Autodesk Fusion 360 part; units mm, degrees
note: some values were not read from the file. Chosen so that the rebuilt part matches the saved one: which face or edge a step refers to. Set by a fixed rule: which sketch regions a step uses.
(part 3 of 7)
  spline S225 degree 3 poles (8.0112, 79.2711) (8.0608, 79.0575) (8.1057, 78.8514) (8.1464, 78.6528) knots 0 0 0 0 1 1 1 1
  spline S226 degree 3 poles (0.8014, 82.2545) (1.2067, 81.299) (1.5221, 80.4293) (1.767, 79.6553) knots 0 0 0 0 1 1 1 1
  arc A227 (1.9503, 79.0495) -> (2.3228, 78.7606) centre (2.3346, 79.1604) ccw
  spline S227 degree 3 poles (4.2579, 78.9588) (4.3292, 79.1486) (4.4058, 79.3452) (4.4881, 79.5484) knots 0 0 0 0 1 1 1 1
  arc A228 (7.2526, 81.938) -> (5.6547, 82.0638) centre (0, 0) ccw
  spline S228 degree 3 poles (-1.9503, 79.0495) (-1.8941, 79.2443) (-1.8331, 79.4462) (-1.767, 79.6553) knots 0 0 0 0 1 1 1 1
  spline S229 degree 3 poles (1.767, 79.6553) (1.8331, 79.4462) (1.8941, 79.2443) (1.9503, 79.0495) knots 0 0 0 0 1 1 1 1
  spline S230 degree 3 poles (19.9812, 79.7947) (20.1522, 78.771) (20.2559, 77.8517) (20.3133, 77.0419) knots 0 0 0 0 1 1 1 1
  spline S231 degree 3 poles (22.5728, 75.7832) (22.6864, 75.9511) (22.8068, 76.1243) (22.9343, 76.3027) knots 0 0 0 0 1 1 1 1
  arc A229 (13.659, 81.1164) -> (12.0759, 81.3672) centre (0, 0) ccw
  spline S232 degree 3 poles (13.659, 81.1164) (13.9098, 80.1093) (14.0853, 79.201) (14.2061, 78.3982) knots 0 0 0 0 1 1 1 1
  spline S233 degree 3 poles (10.7156, 78.951) (11.0785, 79.6772) (11.5261, 80.4868) (12.0759, 81.3672) knots 0 0 0 0 1 1 1 1
  spline S234 degree 3 poles (10.4398, 78.3813) (10.5258, 78.5649) (10.6176, 78.7549) (10.7156, 78.951) knots 0 0 0 0 1 1 1 1
  arc A230 (16.1277, 77.1267) -> (16.5573, 77.3206) centre (16.2095, 77.5182) ccw
  spline S235 degree 3 poles (14.2061, 78.3982) (14.2387, 78.1814) (14.2673, 77.9723) (14.2923, 77.7712) knots 0 0 0 0 1 1 1 1
  spline S236 degree 3 poles (16.5573, 77.3206) (16.6574, 77.4969) (16.7639, 77.6791) (16.877, 77.8669) knots 0 0 0 0 1 1 1 1
  arc A231 (16.1277, 77.1267) -> (14.6151, 77.4275) centre (0, 0) ccw
  arc A232 (14.2923, 77.7712) -> (14.6151, 77.4275) centre (14.6893, 77.8206) ccw
  arc A233 (19.9812, 79.7947) -> (18.4227, 80.1689) centre (0, 0) ccw
  spline S237 degree 3 poles (16.877, 77.8669) (17.2958, 78.5624) (17.8055, 79.3344) (18.4227, 80.1689) knots 0 0 0 0 1 1 1 1
  arc A234 (22.1292, 75.6235) -> (22.5728, 75.7832) centre (22.2416, 76.0074) ccw
  spline S238 degree 3 poles (20.3133, 77.0419) (20.3288, 76.8232) (20.341, 76.6126) (20.3501, 76.41) knots 0 0 0 0 1 1 1 1
  spline S239 degree 3 poles (26.1802, 77.981) (26.2704, 76.9471) (26.3016, 76.0225) (26.2953, 75.2107) knots 0 0 0 0 1 1 1 1
  spline S240 degree 3 poles (22.9343, 76.3027) (23.4064, 76.9632) (23.9752, 77.6928) (24.6558, 78.4763) knots 0 0 0 0 1 1 1 1
  arc A235 (22.1292, 75.6235) -> (20.6449, 76.0422) centre (0, 0) ccw
  spline S241 degree 3 poles (26.2953, 75.2107) (26.2937, 74.9914) (26.2892, 74.7805) (26.2825, 74.5778) knots 0 0 0 0 1 1 1 1
  arc A236 (20.3501, 76.41) -> (20.6449, 76.0422) centre (20.7497, 76.4282) ccw
  arc A237 (26.2825, 74.5778) -> (26.5475, 74.188) centre (26.6822, 74.5646) ccw
  arc A238 (27.9944, 73.6542) -> (28.4491, 73.7785) centre (28.1365, 74.0281) ccw
  arc A239 (26.1802, 77.981) -> (24.6558, 78.4763) centre (0, 0) ccw
  arc A240 (27.9944, 73.6542) -> (26.5475, 74.188) centre (0, 0) ccw
  spline S242 degree 3 poles (28.4491, 73.7785) (28.5755, 73.937) (28.7092, 74.1003) (28.8503, 74.2681) knots 0 0 0 0 1 1 1 1
  spline S243 degree 3 poles (28.8503, 74.2681) (29.3727, 74.8895) (29.997, 75.5723) (30.737, 76.2999) knots 0 0 0 0 1 1 1 1
  arc A241 (32.2178, 75.6865) -> (30.737, 76.2999) centre (0, 0) ccw
  spline S244 degree 3 poles (32.2178, 75.6865) (32.2266, 74.6487) (32.1852, 73.7245) (32.1152, 72.9157) knots 0 0 0 0 1 1 1 1
  arc A242 (33.6869, 71.2307) -> (32.2864, 71.8764) centre (0, 0) ccw
  arc A243 (32.0528, 72.2858) -> (32.2864, 71.8764) centre (32.4503, 72.2413) ccw
  arc A244 (38.0568, 72.9254) -> (36.6287, 73.6531) centre (0, 0) ccw
  spline S245 degree 3 poles (34.15, 71.319) (34.2885, 71.4671) (34.4345, 71.6193) (34.5883, 71.7756) knots 0 0 0 0 1 1 1 1
  arc A245 (37.6254, 69.5482) -> (37.8262, 69.1217) centre (38.0182, 69.4726) ccw
  arc A246 (43.6612, 69.7147) -> (42.2945, 70.5522) centre (0, 0) ccw
  spline S246 degree 3 poles (39.6403, 68.4198) (39.79, 68.5565) (39.9475, 68.6969) (40.1132, 68.8406) knots 0 0 0 0 1 1 1 1
  spline S247 degree 3 poles (43.6612, 69.7147) (43.5075, 68.6883) (43.322, 67.7819) (43.1264, 66.9941) knots 0 0 0 0 1 1 1 1
  spline S248 degree 3 poles (40.1132, 68.8406) (40.7264, 69.3726) (41.4498, 69.9493) (42.2945, 70.5522) knots 0 0 0 0 1 1 1 1
  spline S249 degree 3 poles (32.1152, 72.9157) (32.0964, 72.6972) (32.0754, 72.4873) (32.0528, 72.2858) knots 0 0 0 0 1 1 1 1
  spline S250 degree 3 poles (34.5883, 71.7756) (35.1579, 72.3541) (35.8338, 72.9858) (36.6287, 73.6531) knots 0 0 0 0 1 1 1 1
  spline S251 degree 3 poles (44.8863, 65.0987) (45.0463, 65.2233) (45.2143, 65.3508) (45.3907, 65.4811) knots 0 0 0 0 1 1 1 1
  spline S252 degree 3 poles (37.7371, 70.1712) (37.7012, 69.9549) (37.6638, 69.7473) (37.6254, 69.5482) knots 0 0 0 0 1 1 1 1
  arc A247 (44.4151, 65.084) -> (44.8863, 65.0987) centre (44.6406, 65.4144) ccw
  arc A248 (39.1718, 68.3681) -> (37.8262, 69.1217) centre (0, 0) ccw
  arc A249 (33.6869, 71.2307) -> (34.15, 71.319) centre (33.8579, 71.5923) ccw
  arc A250 (39.1718, 68.3681) -> (39.6403, 68.4198) centre (39.3706, 68.7152) ccw
  spline S253 degree 3 poles (43.1264, 66.9941) (43.0736, 66.7812) (43.02, 66.5772) (42.9661, 66.3817) knots 0 0 0 0 1 1 1 1
  arc A251 (44.4151, 65.084) -> (43.1328, 65.9408) centre (0, 0) ccw
  arc A252 (42.9661, 66.3817) -> (43.1328, 65.9408) centre (43.3518, 66.2755) ccw
  spline S254 degree 3 poles (38.0568, 72.9254) (37.9841, 71.8901) (37.8704, 70.972) (37.7371, 70.1712) knots 0 0 0 0 1 1 1 1
  spline S255 degree 3 poles (45.3907, 65.4811) (46.0437, 65.9633) (46.8101, 66.4815) (47.6996, 67.0163) knots 0 0 0 0 1 1 1 1
  spline S256 degree 3 poles (50.3883, 61.7179) (51.0772, 62.1475) (51.8819, 62.6039) (52.8106, 63.0673) knots 0 0 0 0 1 1 1 1
  spline S257 degree 3 poles (54.0294, 62.0263) (53.717, 61.0366) (53.3921, 60.1704) (53.0756, 59.4228) knots 0 0 0 0 1 1 1 1
  arc A253 (52.8215, 58.8431) -> (52.9172, 58.3815) centre (53.1858, 58.6778) ccw
  spline S258 degree 3 poles (49.8555, 61.3763) (50.0247, 61.4879) (50.2023, 61.6019) (50.3883, 61.7179) knots 0 0 0 0 1 1 1 1
  arc A254 (58.7294, 57.596) -> (57.596, 58.7294) centre (0, 0) ccw
  spline S259 degree 3 poles (48.9963, 66.0742) (48.7626, 65.063) (48.5066, 64.174) (48.2497, 63.4039) knots 0 0 0 0 1 1 1 1
  arc A255 (49.3846, 61.3986) -> (48.1735, 62.3533) centre (0, 0) ccw
  arc A256 (54.0497, 57.3346) -> (54.5174, 57.2755) centre (54.324, 57.6257) ccw
  arc A257 (48.0419, 62.806) -> (48.1735, 62.3533) centre (48.418, 62.6699) ccw
  spline S260 degree 3 poles (55.0753, 57.5742) (55.7958, 57.9484) (56.6338, 58.3403) (57.596, 58.7294) knots 0 0 0 0 1 1 1 1
  arc A258 (54.0497, 57.3346) -> (52.9172, 58.3815) centre (0, 0) ccw
  arc A259 (54.0294, 62.0263) -> (52.8106, 63.0673) centre (0, 0) ccw
  spline S261 degree 3 poles (54.5174, 57.2755) (54.6948, 57.3735) (54.8807, 57.4732) (55.0753, 57.5742) knots 0 0 0 0 1 1 1 1
  spline S262 degree 3 poles (53.0756, 59.4228) (52.9901, 59.2209) (52.9053, 59.0277) (52.8215, 58.8431) knots 0 0 0 0 1 1 1 1
  arc A260 (49.3846, 61.3986) -> (49.8555, 61.3763) centre (49.6353, 61.7102) ccw
  spline S263 degree 3 poles (48.2497, 63.4039) (48.1804, 63.1959) (48.111, 62.9966) (48.0419, 62.806) knots 0 0 0 0 1 1 1 1
  spline S264 degree 3 poles (57.5742, 55.0753) (57.4732, 54.8807) (57.3735, 54.6948) (57.2755, 54.5174) knots 0 0 0 0 1 1 1 1
  arc A261 (48.9963, 66.0742) -> (47.6996, 67.0163) centre (0, 0) ccw
  arc A262 (58.3815, 52.9172) -> (57.3346, 54.0497) centre (0, 0) ccw
  arc A263 (58.3815, 52.9172) -> (58.8431, 52.8215) centre (58.6778, 53.1858) ccw
  spline S265 degree 3 poles (59.4228, 53.0756) (60.1704, 53.3921) (61.0366, 53.717) (62.0263, 54.0294) knots 0 0 0 0 1 1 1 1
  spline S266 degree 3 poles (58.7294, 57.596) (58.3403, 56.6338) (57.9484, 55.7958) (57.5742, 55.0753) knots 0 0 0 0 1 1 1 1
  arc A264 (63.0673, 52.8106) -> (62.0263, 54.0294) centre (0, 0) ccw
  arc A265 (57.2755, 54.5174) -> (57.3346, 54.0497) centre (57.6257, 54.324) ccw
  spline S267 degree 3 poles (58.8431, 52.8215) (59.0277, 52.9053) (59.2209, 52.9901) (59.4228, 53.0756) knots 0 0 0 0 1 1 1 1
  spline S268 degree 3 poles (62.806, 48.0419) (62.9966, 48.111) (63.1959, 48.1804) (63.4039, 48.2497) knots 0 0 0 0 1 1 1 1
  arc A266 (62.3533, 48.1735) -> (61.3986, 49.3846) centre (0, 0) ccw
  arc A267 (62.3533, 48.1735) -> (62.806, 48.0419) centre (62.6699, 48.418) ccw
  spline S269 degree 3 poles (67.0163, 47.6996) (66.4815, 46.8101) (65.9633, 46.0437) (65.4811, 45.3907) knots 0 0 0 0 1 1 1 1
  spline S270 degree 3 poles (63.4039, 48.2497) (64.174, 48.5066) (65.063, 48.7626) (66.0742, 48.9963) knots 0 0 0 0 1 1 1 1
  arc A268 (67.0163, 47.6996) -> (66.0742, 48.9963) centre (0, 0) ccw
  spline S271 degree 3 poles (63.0673, 52.8106) (62.6039, 51.8819) (62.1475, 51.0772) (61.7179, 50.3883) knots 0 0 0 0 1 1 1 1
  spline S272 degree 3 poles (61.7179, 50.3883) (61.6019, 50.2023) (61.4879, 50.0247) (61.3763, 49.8555) knots 0 0 0 0 1 1 1 1
  arc A269 (61.3763, 49.8555) -> (61.3986, 49.3846) centre (61.7102, 49.6353) ccw
  arc A270 (65.9408, 43.1328) -> (65.084, 44.4151) centre (0, 0) ccw
  arc A271 (65.0987, 44.8863) -> (65.084, 44.4151) centre (65.4144, 44.6406) ccw
  spline S273 degree 3 poles (66.3817, 42.9661) (66.5772, 43.02) (66.7812, 43.0736) (66.9941, 43.1264) knots 0 0 0 0 1 1 1 1
  spline S274 degree 3 poles (65.4811, 45.3907) (65.3508, 45.2143) (65.2233, 45.0463) (65.0987, 44.8863) knots 0 0 0 0 1 1 1 1
  arc A272 (70.5522, 42.2945) -> (69.7147, 43.6612) centre (0, 0) ccw
  arc A273 (73.6531, 36.6287) -> (72.9254, 38.0568) centre (0, 0) ccw
  spline S275 degree 3 poles (68.8406, 40.1132) (68.6969, 39.9475) (68.5565, 39.79) (68.4198, 39.6403) knots 0 0 0 0 1 1 1 1
  spline S276 degree 3 poles (70.1712, 37.7371) (70.972, 37.8704) (71.8901, 37.9841) (72.9254, 38.0568) knots 0 0 0 0 1 1 1 1
  arc A274 (-2.3228, 78.7606) -> (-1.9503, 79.0495) centre (-2.3346, 79.1604) ccw
  spline S277 degree 3 poles (70.5522, 42.2945) (69.9493, 41.4498) (69.3726, 40.7264) (68.8406, 40.1132) knots 0 0 0 0 1 1 1 1
  arc A275 (68.4198, 39.6403) -> (68.3681, 39.1718) centre (68.7152, 39.3706) ccw
  spline S278 degree 3 poles (-4.4881, 79.5484) (-4.4058, 79.3452) (-4.3292, 79.1486) (-4.2579, 78.9588) knots 0 0 0 0 1 1 1 1
  arc A276 (65.9408, 43.1328) -> (66.3817, 42.9661) centre (66.2755, 43.3518) ccw
  arc A277 (-2.3228, 78.7606) -> (-3.8638, 78.7) centre (0, 0) ccw
  spline S279 degree 3 poles (-5.6547, 82.0638) (-5.1757, 81.1431) (-4.793, 80.3008) (-4.4881, 79.5484) knots 0 0 0 0 1 1 1 1
  arc A278 (-4.2579, 78.9588) -> (-3.8638, 78.7) centre (-3.8835, 79.0995) ccw
  spline S280 degree 3 poles (66.9941, 43.1264) (67.7819, 43.322) (68.6883, 43.5075) (69.7147, 43.6612) knots 0 0 0 0 1 1 1 1
  spline S281 degree 3 poles (69.5482, 37.6254) (69.7473, 37.6638) (69.9549, 37.7012) (70.1712, 37.7371) knots 0 0 0 0 1 1 1 1
  arc A279 (69.1217, 37.8262) -> (69.5482, 37.6254) centre (69.4726, 38.0182) ccw
  arc A280 (69.1217, 37.8262) -> (68.3681, 39.1718) centre (0, 0) ccw
  spline S282 degree 3 poles (73.6531, 36.6287) (72.9858, 35.8338) (72.3541, 35.1579) (71.7756, 34.5883) knots 0 0 0 0 1 1 1 1
  spline S283 degree 3 poles (72.2858, 32.0528) (72.4873, 32.0754) (72.6972, 32.0964) (72.9157, 32.1152) knots 0 0 0 0 1 1 1 1
  spline S284 degree 3 poles (76.2999, 30.737) (75.5723, 29.997) (74.8895, 29.3727) (74.2681, 28.8503) knots 0 0 0 0 1 1 1 1
  spline S285 degree 3 poles (74.5778, 26.2825) (74.7805, 26.2892) (74.9914, 26.2937) (75.2107, 26.2953) knots 0 0 0 0 1 1 1 1
  spline S286 degree 3 poles (76.41, 20.3501) (76.6126, 20.341) (76.8232, 20.3288) (77.0419, 20.3133) knots 0 0 0 0 1 1 1 1
  spline S287 degree 3 poles (71.7756, 34.5883) (71.6193, 34.4345) (71.4671, 34.2885) (71.319, 34.15) knots 0 0 0 0 1 1 1 1
  arc A281 (73.7785, 28.4491) -> (73.6542, 27.9944) centre (74.0281, 28.1365) ccw
  arc A282 (71.319, 34.15) -> (71.2307, 33.6869) centre (71.5923, 33.8579) ccw
  arc A283 (74.188, 26.5475) -> (73.6542, 27.9944) centre (0, 0) ccw
  spline S288 degree 3 poles (74.2681, 28.8503) (74.1003, 28.7092) (73.937, 28.5755) (73.7785, 28.4491) knots 0 0 0 0 1 1 1 1
  arc A284 (74.188, 26.5475) -> (74.5778, 26.2825) centre (74.5646, 26.6822) ccw
  arc A285 (76.2999, 30.737) -> (75.6865, 32.2178) centre (0, 0) ccw
  arc A286 (71.8764, 32.2864) -> (71.2307, 33.6869) centre (0, 0) ccw
  arc A287 (71.8764, 32.2864) -> (72.2858, 32.0528) centre (72.2413, 32.4503) ccw
  spline S289 degree 3 poles (72.9157, 32.1152) (73.7245, 32.1852) (74.6487, 32.2266) (75.6865, 32.2178) knots 0 0 0 0 1 1 1 1
  spline S290 degree 3 poles (76.3027, 22.9343) (76.1243, 22.8068) (75.9511, 22.6864) (75.7832, 22.5728) knots 0 0 0 0 1 1 1 1
  spline S291 degree 3 poles (75.2107, 26.2953) (76.0225, 26.3016) (76.9471, 26.2704) (77.981, 26.1802) knots 0 0 0 0 1 1 1 1
  arc A288 (75.7832, 22.5728) -> (75.6235, 22.1292) centre (76.0074, 22.2416) ccw
  spline S292 degree 3 poles (80.1689, 18.4227) (79.3344, 17.8055) (78.5624, 17.2958) (77.8669, 16.877) knots 0 0 0 0 1 1 1 1
  arc A289 (77.4275, 14.6151) -> (77.1267, 16.1277) centre (0, 0) ccw
  spline S293 degree 3 poles (78.4763, 24.6558) (77.6928, 23.9752) (76.9632, 23.4064) (76.3027, 22.9343) knots 0 0 0 0 1 1 1 1
  arc A290 (78.4763, 24.6558) -> (77.981, 26.1802) centre (0, 0) ccw
  arc A291 (76.0422, 20.6449) -> (76.41, 20.3501) centre (76.4282, 20.7497) ccw
  arc A292 (76.0422, 20.6449) -> (75.6235, 22.1292) centre (0, 0) ccw
  arc A293 (77.3206, 16.5573) -> (77.1267, 16.1277) centre (77.5182, 16.2095) ccw
  spline S294 degree 3 poles (77.8669, 16.877) (77.6791, 16.7639) (77.4969, 16.6574) (77.3206, 16.5573) knots 0 0 0 0 1 1 1 1
  spline S295 degree 3 poles (77.0419, 20.3133) (77.8517, 20.2559) (78.771, 20.1522) (79.7947, 19.9812) knots 0 0 0 0 1 1 1 1
  arc A294 (80.1689, 18.4227) -> (79.7947, 19.9812) centre (0, 0) ccw
  spline S296 degree 3 poles (77.7712, 14.2923) (77.9723, 14.2673) (78.1814, 14.2387) (78.3982, 14.2061) knots 0 0 0 0 1 1 1 1
  arc A295 (78.3355, 8.4951) -> (78.6528, 8.1464) centre (78.7332, 8.5383) ccw
  spline S297 degree 3 poles (81.3672, 12.0759) (80.4868, 11.5261) (79.6772, 11.0785) (78.951, 10.7156) knots 0 0 0 0 1 1 1 1
  arc A296 (81.3672, 12.0759) -> (81.1164, 13.659) centre (0, 0) ccw
  spline S298 degree 3 poles (78.3982, 14.2061) (79.201, 14.0853) (80.1093, 13.9098) (81.1164, 13.659) knots 0 0 0 0 1 1 1 1
  arc A297 (77.4275, 14.6151) -> (77.7712, 14.2923) centre (77.8206, 14.6893) ccw
  arc A298 (78.3813, 10.4398) -> (78.1543, 10.0267) centre (78.551, 10.0776) ccw
  arc A299 (78.3355, 8.4951) -> (78.1543, 10.0267) centre (0, 0) ccw
  spline S299 degree 3 poles (79.2711, 8.0112) (80.0619, 7.8278) (80.9537, 7.5816) (81.938, 7.2526) knots 0 0 0 0 1 1 1 1
  spline S300 degree 3 poles (79.5484, 4.4881) (79.3452, 4.4058) (79.1486, 4.3292) (78.9588, 4.2579) knots 0 0 0 0 1 1 1 1
  spline S301 degree 3 poles (78.951, 10.7156) (78.7549, 10.6176) (78.5649, 10.5258) (78.3813, 10.4398) knots 0 0 0 0 1 1 1 1
  spline S302 degree 3 poles (82.0638, 5.6547) (81.1431, 5.1757) (80.3008, 4.793) (79.5484, 4.4881) knots 0 0 0 0 1 1 1 1
  spline S303 degree 3 poles (82.2545, -0.8014) (81.299, -1.2067) (80.4293, -1.5221) (79.6553, -1.767) knots 0 0 0 0 1 1 1 1
  arc A300 (78.7606, 2.3228) -> (79.0495, 1.9503) centre (79.1604, 2.3346) ccw
  arc A301 (78.7606, 2.3228) -> (78.7, 3.8638) centre (0, 0) ccw
  arc A302 (78.9588, 4.2579) -> (78.7, 3.8638) centre (79.0995, 3.8835) ccw
  arc A303 (82.0638, 5.6547) -> (81.938, 7.2526) centre (0, 0) ccw
  spline S304 degree 3 poles (78.6528, 8.1464) (78.8514, 8.1057) (79.0575, 8.0608) (79.2711, 8.0112) knots 0 0 0 0 1 1 1 1
  spline S305 degree 3 poles (79.6553, 1.767) (80.4293, 1.5221) (81.299, 1.2067) (82.2545, 0.8014) knots 0 0 0 0 1 1 1 1
  spline S306 degree 3 poles (79.0495, 1.9503) (79.2443, 1.8941) (79.4462, 1.8331) (79.6553, 1.767) knots 0 0 0 0 1 1 1 1
  arc A304 (82.2545, -0.8014) -> (82.2545, 0.8014) centre (0, 0) ccw
  arc A305 (79.0495, -1.9503) -> (78.7606, -2.3228) centre (79.1604, -2.3346) ccw
  spline S307 degree 3 poles (79.6553, -1.767) (79.4462, -1.8331) (79.2443, -1.8941) (79.0495, -1.9503) knots 0 0 0 0 1 1 1 1
  arc A306 (76.41, -20.3501) -> (76.0422, -20.6449) centre (76.4282, -20.7497) ccw
  arc A307 (75.6235, -22.1292) -> (76.0422, -20.6449) centre (0, 0) ccw
  spline S308 degree 3 poles (77.0419, -20.3133) (76.8232, -20.3288) (76.6126, -20.341) (76.41, -20.3501) knots 0 0 0 0 1 1 1 1
  arc A308 (78.7, -3.8638) -> (78.9588, -4.2579) centre (79.0995, -3.8835) ccw
  arc A309 (78.1543, -10.0267) -> (78.3355, -8.4951) centre (0, 0) ccw
  arc A310 (78.6528, -8.1464) -> (78.3355, -8.4951) centre (78.7332, -8.5383) ccw
  spline S309 degree 3 poles (81.938, -7.2526) (80.9537, -7.5816) (80.0619, -7.8278) (79.2711, -8.0112) knots 0 0 0 0 1 1 1 1
  circle A311 centre (0, 0) radius 92.5
  spline S310 degree 3 poles (78.9588, -4.2579) (79.1486, -4.3292) (79.3452, -4.4058) (79.5484, -4.4881) knots 0 0 0 0 1 1 1 1
  arc A312 (78.7, -3.8638) -> (78.7606, -2.3228) centre (0, 0) ccw
  arc A313 (75.6235, -22.1292) -> (75.7832, -22.5728) centre (76.0074, -22.2416) ccw
  arc A314 (77.7712, -14.2923) -> (77.4275, -14.6151) centre (77.8206, -14.6893) ccw
  spline S311 degree 3 poles (78.3813, -10.4398) (78.5649, -10.5258) (78.7549, -10.6176) (78.951, -10.7156) knots 0 0 0 0 1 1 1 1
  arc A315 (81.938, -7.2526) -> (82.0638, -5.6547) centre (0, 0) ccw
  spline S312 degree 3 poles (79.5484, -4.4881) (80.3008, -4.793) (81.1431, -5.1757) (82.0638, -5.6547) knots 0 0 0 0 1 1 1 1
  spline S313 degree 3 poles (79.2711, -8.0112) (79.0575, -8.0608) (78.8514, -8.1057) (78.6528, -8.1464) knots 0 0 0 0 1 1 1 1
  arc A316 (77.1267, -16.1277) -> (77.3206, -16.5573) centre (77.5182, -16.2095) ccw
  spline S314 degree 3 poles (78.3982, -14.2061) (78.1814, -14.2387) (77.9723, -14.2673) (77.7712, -14.2923) knots 0 0 0 0 1 1 1 1
  arc A317 (81.1164, -13.659) -> (81.3672, -12.0759) centre (0, 0) ccw
  arc A318 (78.1543, -10.0267) -> (78.3813, -10.4398) centre (78.551, -10.0776) ccw
  arc A319 (77.1267, -16.1277) -> (77.4275, -14.6151) centre (0, 0) ccw
  spline S315 degree 3 poles (78.951, -10.7156) (79.6772, -11.0785) (80.4868, -11.5261) (81.3672, -12.0759) knots 0 0 0 0 1 1 1 1
  spline S316 degree 3 poles (77.3206, -16.5573) (77.4969, -16.6574) (77.6791, -16.7639) (77.8669, -16.877) knots 0 0 0 0 1 1 1 1
  spline S317 degree 3 poles (81.1164, -13.659) (80.1093, -13.9098) (79.201, -14.0853) (78.3982, -14.2061) knots 0 0 0 0 1 1 1 1
  spline S318 degree 3 poles (77.8669, -16.877) (78.5624, -17.2958) (79.3344, -17.8055) (80.1689, -18.4227) knots 0 0 0 0 1 1 1 1
  spline S319 degree 3 poles (79.7947, -19.9812) (78.771, -20.1522) (77.8517, -20.2559) (77.0419, -20.3133) knots 0 0 0 0 1 1 1 1
  arc A320 (79.7947, -19.9812) -> (80.1689, -18.4227) centre (0, 0) ccw
extrude "Extrude1''" add sketch "sketch 33723" along normal blind 8 separate body makes body 3 in component "Internal Gear (80 teeth)"
sketch "Sketch1 (3)" plane through (0, 0, 0) normal (0, 1, 0) x (1, 0, 0) in component "Internal Gear (80 teeth)"
  circle A0 centre (0, 0) radius 80.252 construction
sketch "Sketch13" plane through (0, 0, 0) normal (0, -1, 0) x (1, 0, 0)
  circle A0 centre (41.6795, 43.1604) radius 12.5
  line L0 (32.6264, 59.9389) -> (33.0778, 59.1022)
  arc A1 (32.9235, 58.5645) -> (33.0778, 59.1022) centre (32.7258, 58.9122) ccw
  arc A2 (32.9235, 58.5645) -> (31.6728, 57.783) centre (41.6795, 43.1604) ccw
  arc A3 (31.1218, 57.8799) -> (31.6728, 57.783) centre (31.4469, 58.1131) ccw
  line L1 (31.1218, 57.8799) -> (30.5677, 58.6525)
  spline S0 degree 3 poles (29.9216, 59.2371) (30.3165, 58.9424) (30.5073, 58.7267) (30.5677, 58.6525) knots 0 0 0 0 1 1 1 1
  spline S1 degree 3 poles (27.602, 60.4259) (28.704, 60.0341) (29.4506, 59.5874) (29.9216, 59.2371) knots 0 0 0 0 1 1 1 1
  arc A4 (27.602, 60.4259) -> (26.5412, 59.5038) centre (41.6795, 43.1604) ccw
  spline S2 degree 3 poles (27.3959, 57.04) (27.1142, 57.5565) (26.7758, 58.358) (26.5412, 59.5038) knots 0 0 0 0 1 1 1 1
  spline S3 degree 3 poles (27.8846, 56.3201) (27.8195, 56.3903) (27.6325, 56.6092) (27.3959, 57.04) knots 0 0 0 0 1 1 1 1
  line L2 (27.8846, 56.3201) -> (28.5725, 55.6639)
  arc A5 (28.5919, 55.1048) -> (28.5725, 55.6639) centre (28.2964, 55.3744) ccw
  arc A6 (28.5919, 55.1048) -> (27.6439, 53.975) centre (41.6795, 43.1604) ccw
  arc A7 (27.09, 53.897) -> (27.6439, 53.975) centre (27.3271, 54.2192) ccw
  line L3 (27.09, 53.897) -> (26.3242, 54.4605)
  spline S4 degree 3 poles (25.5291, 54.8168) (25.9958, 54.6586) (26.2438, 54.5124) (26.3242, 54.4605) knots 0 0 0 0 1 1 1 1
  spline S5 degree 3 poles (22.9557, 55.2307) (24.1248, 55.1986) (24.9729, 55.0045) (25.5291, 54.8168) knots 0 0 0 0 1 1 1 1
  arc A8 (22.9557, 55.2307) -> (22.2317, 54.0259) centre (41.6795, 43.1604) ccw
  spline S6 degree 3 poles (23.8059, 51.9468) (23.3785, 52.351) (22.8089, 53.0087) (22.2317, 54.0259) knots 0 0 0 0 1 1 1 1
  spline S7 degree 3 poles (24.4932, 51.4132) (24.4096, 51.4598) (24.1641, 51.6102) (23.8059, 51.9468) knots 0 0 0 0 1 1 1 1
  line L4 (24.4932, 51.4132) -> (25.3503, 51.0016)
  arc A9 (25.5414, 50.4759) -> (25.3503, 51.0016) centre (25.1771, 50.641) ccw
  arc A10 (25.5414, 50.4759) -> (24.989, 49.1085) centre (41.6795, 43.1604) ccw
  arc A11 (24.4862, 48.8631) -> (24.989, 49.1085) centre (24.6122, 49.2428) ccw
  line L5 (24.4862, 48.8631) -> (23.5838, 49.1624)
  spline S8 degree 3 poles (22.7175, 49.2556) (23.2102, 49.2493) (23.4913, 49.1869) (23.5838, 49.1624) knots 0 0 0 0 1 1 1 1
  spline S9 degree 3 poles (20.1421, 48.854) (21.264, 49.1847) (22.1305, 49.2622) (22.7175, 49.2556) knots 0 0 0 0 1 1 1 1
  arc A12 (20.1421, 48.854) -> (19.826, 47.4844) centre (41.6795, 43.1604) ccw
  spline S10 degree 3 poles (21.9656, 45.9935) (21.4341, 46.2458) (20.6892, 46.6953) (19.826, 47.4844) knots 0 0 0 0 1 1 1 1
  spline S11 degree 3 poles (22.7841, 45.6984) (22.6902, 45.7169) (22.4102, 45.7841) (21.9656, 45.9935) knots 0 0 0 0 1 1 1 1
  line L6 (22.7841, 45.6984) -> (23.7264, 45.5718)
  arc A13 (24.0707, 45.1309) -> (23.7264, 45.5718) centre (23.6731, 45.1754) ccw
  arc A14 (24.0707, 45.1309) -> (23.9678, 43.6597) centre (41.6795, 43.1604) ccw
  arc A15 (23.5655, 43.271) -> (23.9678, 43.6597) centre (23.5679, 43.671) ccw
  line L7 (23.5655, 43.271) -> (22.6148, 43.2768)
  spline S12 degree 3 poles (21.7621, 43.0977) (22.2326, 43.2439) (22.5192, 43.2715) (22.6148, 43.2768) knots 0 0 0 0 1 1 1 1
  spline S13 degree 3 poles (19.4368, 41.9199) (20.4016, 42.5811) (21.2017, 42.9226) (21.7621, 43.0977) knots 0 0 0 0 1 1 1 1
  arc A16 (19.4368, 41.9199) -> (19.5594, 40.5196) centre (41.6795, 43.1604) ccw
  spline S14 degree 3 poles (22.055, 39.7629) (21.4715, 39.8387) (20.6242, 40.036) (19.5594, 40.5196) knots 0 0 0 0 1 1 1 1
  spline S15 degree 3 poles (22.9246, 39.7352) (22.8296, 39.7238) (22.5426, 39.7012) (22.055, 39.7629) knots 0 0 0 0 1 1 1 1
  line L8 (22.9246, 39.7352) -> (23.8599, 39.906)
  arc A17 (24.3236, 39.593) -> (23.8599, 39.906) centre (23.9318, 39.5125) ccw
  arc A18 (24.3236, 39.593) -> (24.6804, 38.1621) centre (41.6795, 43.1604) ccw
  arc A19 (24.4179, 37.6681) -> (24.6804, 38.1621) centre (24.2966, 38.0492) ccw
  line L9 (24.4179, 37.6681) -> (23.5119, 37.3798)
  spline S16 degree 3 poles (22.7563, 36.9459) (23.1586, 37.2304) (23.4226, 37.3452) (23.5119, 37.3798) knots 0 0 0 0 1 1 1 1
  spline S17 degree 3 poles (20.9088, 35.1072) (21.622, 36.0342) (22.2775, 36.6062) (22.7563, 36.9459) knots 0 0 0 0 1 1 1 1
  arc A20 (20.9088, 35.1072) -> (21.458, 33.8134) centre (41.6795, 43.1604) ccw
  spline S18 degree 3 poles (24.0654, 33.8649) (23.4871, 33.7566) (22.6202, 33.6825) (21.458, 33.8134) knots 0 0 0 0 1 1 1 1
  spline S19 degree 3 poles (24.901, 34.1072) (24.8141, 34.0671) (24.5482, 33.9568) (24.0654, 33.8649) knots 0 0 0 0 1 1 1 1
  line L10 (24.901, 34.1072) -> (25.7377, 34.5587)
  arc A21 (26.2754, 34.4044) -> (25.7377, 34.5587) centre (25.9277, 34.2067) ccw
  arc A22 (26.2754, 34.4044) -> (27.0569, 33.1537) centre (41.6795, 43.1604) ccw
  arc A23 (26.96, 32.6027) -> (27.0569, 33.1537) centre (26.7268, 32.9278) ccw
  line L11 (26.96, 32.6027) -> (26.1874, 32.0486)
  spline S20 degree 3 poles (25.6028, 31.4025) (25.8975, 31.7974) (26.1132, 31.9882) (26.1874, 32.0486) knots 0 0 0 0 1 1 1 1
  spline S21 degree 3 poles (24.414, 29.0829) (24.8058, 30.1849) (25.2524, 30.9315) (25.6028, 31.4025) knots 0 0 0 0 1 1 1 1
  arc A24 (24.414, 29.0829) -> (25.3361, 28.0221) centre (41.6795, 43.1604) ccw
  spline S22 degree 3 poles (27.7999, 28.8768) (27.2834, 28.5951) (26.4819, 28.2567) (25.3361, 28.0221) knots 0 0 0 0 1 1 1 1
  spline S23 degree 3 poles (28.5198, 29.3655) (28.4496, 29.3004) (28.2307, 29.1134) (27.7999, 28.8768) knots 0 0 0 0 1 1 1 1
  line L12 (28.5198, 29.3655) -> (29.176, 30.0534)
  arc A25 (29.7351, 30.0728) -> (29.176, 30.0534) centre (29.4655, 29.7773) ccw
  arc A26 (29.7351, 30.0728) -> (30.8648, 29.1248) centre (41.6795, 43.1604) ccw
  arc A27 (30.9429, 28.5709) -> (30.8648, 29.1248) centre (30.6207, 28.808) ccw
  line L13 (30.9429, 28.5709) -> (30.3793, 27.8051)
  spline S24 degree 3 poles (30.0231, 27.01) (30.1813, 27.4766) (30.3275, 27.7247) (30.3793, 27.8051) knots 0 0 0 0 1 1 1 1
  spline S25 degree 3 poles (29.6092, 24.4366) (29.6413, 25.6057) (29.8354, 26.4537) (30.0231, 27.01) knots 0 0 0 0 1 1 1 1
  arc A28 (29.6092, 24.4366) -> (30.814, 23.7126) centre (41.6795, 43.1604) ccw
  spline S26 degree 3 poles (32.8931, 25.2868) (32.4889, 24.8594) (31.8312, 24.2898) (30.814, 23.7126) knots 0 0 0 0 1 1 1 1
  spline S27 degree 3 poles (33.4267, 25.9741) (33.3801, 25.8905) (33.2297, 25.645) (32.8931, 25.2868) knots 0 0 0 0 1 1 1 1
  line L14 (33.4267, 25.9741) -> (33.8383, 26.8311)
  arc A29 (34.364, 27.0223) -> (33.8383, 26.8311) centre (34.1988, 26.658) ccw
  arc A30 (34.364, 27.0223) -> (35.7314, 26.4698) centre (41.6795, 43.1604) ccw
  arc A31 (35.9768, 25.9671) -> (35.7314, 26.4698) centre (35.5971, 26.0931) ccw
  line L15 (35.9768, 25.9671) -> (35.6775, 25.0647)
  spline S28 degree 3 poles (35.5843, 24.1984) (35.5906, 24.6911) (35.653, 24.9722) (35.6775, 25.0647) knots 0 0 0 0 1 1 1 1
  spline S29 degree 3 poles (35.9859, 21.623) (35.6552, 22.7448) (35.5777, 23.6114) (35.5843, 24.1984) knots 0 0 0 0 1 1 1 1
  arc A32 (35.9859, 21.623) -> (37.3555, 21.3068) centre (41.6795, 43.1604) ccw
  spline S30 degree 3 poles (38.8464, 23.4465) (38.594, 22.915) (38.1445, 22.1701) (37.3555, 21.3068) knots 0 0 0 0 1 1 1 1
  spline S31 degree 3 poles (39.1415, 24.265) (39.123, 24.1711) (39.0558, 23.8911) (38.8464, 23.4465) knots 0 0 0 0 1 1 1 1
  line L16 (39.1415, 24.265) -> (39.2681, 25.2073)
  arc A33 (39.709, 25.5515) -> (39.2681, 25.2073) centre (39.6645, 25.154) ccw
  arc A34 (39.709, 25.5515) -> (41.1802, 25.4487) centre (41.6795, 43.1604) ccw
  arc A35 (41.5689, 25.0464) -> (41.1802, 25.4487) centre (41.1689, 25.0488) ccw
  line L17 (41.5689, 25.0464) -> (41.5631, 24.0957)
  spline S32 degree 3 poles (41.7422, 23.243) (41.5959, 23.7135) (41.5684, 24.0001) (41.5631, 24.0957) knots 0 0 0 0 1 1 1 1
  spline S33 degree 3 poles (42.92, 20.9177) (42.2588, 21.8824) (41.9173, 22.6826) (41.7422, 23.243) knots 0 0 0 0 1 1 1 1
  arc A36 (42.92, 20.9177) -> (44.3202, 21.0402) centre (41.6795, 43.1604) ccw
  spline S34 degree 3 poles (45.077, 23.5359) (45.0012, 22.9524) (44.8039, 22.1051) (44.3202, 21.0402) knots 0 0 0 0 1 1 1 1
  spline S35 degree 3 poles (45.1047, 24.4055) (45.1161, 24.3105) (45.1387, 24.0235) (45.077, 23.5359) knots 0 0 0 0 1 1 1 1
  line L18 (45.1047, 24.4055) -> (44.9339, 25.3408)
  arc A37 (45.2469, 25.8045) -> (44.9339, 25.3408) centre (45.3274, 25.4127) ccw
  arc A38 (45.2469, 25.8045) -> (46.6778, 26.1612) centre (41.6795, 43.1604) ccw
  arc A39 (47.1718, 25.8988) -> (46.6778, 26.1612) centre (46.7907, 25.7775) ccw
  line L19 (47.1718, 25.8988) -> (47.4601, 24.9928)
  spline S36 degree 3 poles (47.894, 24.2372) (47.6094, 24.6395) (47.4947, 24.9035) (47.4601, 24.9928) knots 0 0 0 0 1 1 1 1
  spline S37 degree 3 poles (49.7326, 22.3897) (48.8057, 23.1029) (48.2337, 23.7584) (47.894, 24.2372) knots 0 0 0 0 1 1 1 1
  arc A40 (49.7326, 22.3897) -> (51.0265, 22.9389) centre (41.6795, 43.1604) ccw
  spline S38 degree 3 poles (50.975, 25.5462) (51.0832, 24.9679) (51.1574, 24.1011) (51.0265, 22.9389) knots 0 0 0 0 1 1 1 1
  spline S39 degree 3 poles (50.7326, 26.3819) (50.7728, 26.295) (50.883, 26.029) (50.975, 25.5462) knots 0 0 0 0 1 1 1 1
  line L20 (50.7326, 26.3819) -> (50.2812, 27.2186)
  arc A41 (50.4355, 27.7563) -> (50.2812, 27.2186) centre (50.6332, 27.4085) ccw
  arc A42 (50.4355, 27.7563) -> (51.6862, 28.5378) centre (41.6795, 43.1604) ccw
  arc A43 (52.2372, 28.4408) -> (51.6862, 28.5378) centre (51.9121, 28.2077) ccw
  line L21 (52.2372, 28.4408) -> (52.7913, 27.6683)
  spline S40 degree 3 poles (53.4374, 27.0837) (53.0425, 27.3784) (52.8517, 27.5941) (52.7913, 27.6683) knots 0 0 0 0 1 1 1 1
  spline S41 degree 3 poles (55.757, 25.8948) (54.655, 26.2867) (53.9084, 26.7333) (53.4374, 27.0837) knots 0 0 0 0 1 1 1 1
  arc A44 (55.757, 25.8948) -> (56.8178, 26.817) centre (41.6795, 43.1604) ccw
  spline S42 degree 3 poles (55.9631, 29.2808) (56.2448, 28.7643) (56.5832, 27.9628) (56.8178, 26.817) knots 0 0 0 0 1 1 1 1
  spline S43 degree 3 poles (55.4744, 30.0007) (55.5395, 29.9305) (55.7265, 29.7116) (55.9631, 29.2808) knots 0 0 0 0 1 1 1 1
  line L22 (55.4744, 30.0007) -> (54.7865, 30.6569)
  arc A45 (54.7671, 31.216) -> (54.7865, 30.6569) centre (55.0626, 30.9463) ccw
  arc A46 (54.7671, 31.216) -> (55.7151, 32.3457) centre (41.6795, 43.1604) ccw
  arc A47 (56.269, 32.4238) -> (55.7151, 32.3457) centre (56.0319, 32.1016) ccw
  line L23 (56.269, 32.4238) -> (57.0348, 31.8602)
  spline S44 degree 3 poles (57.8299, 31.504) (57.3632, 31.6622) (57.1152, 31.8083) (57.0348, 31.8602) knots 0 0 0 0 1 1 1 1
  spline S45 degree 3 poles (60.4033, 31.0901) (59.2342, 31.1222) (58.3861, 31.3163) (57.8299, 31.504) knots 0 0 0 0 1 1 1 1
  arc A48 (60.4033, 31.0901) -> (61.1273, 32.2949) centre (41.6795, 43.1604) ccw
  spline S46 degree 3 poles (59.5531, 34.374) (59.9805, 33.9698) (60.5501, 33.3121) (61.1273, 32.2949) knots 0 0 0 0 1 1 1 1
  spline S47 degree 3 poles (58.8658, 34.9076) (58.9494, 34.861) (59.1949, 34.7105) (59.5531, 34.374) knots 0 0 0 0 1 1 1 1
  line L24 (58.8658, 34.9076) -> (58.0087, 35.3192)
  arc A49 (57.8176, 35.8449) -> (58.0087, 35.3192) centre (58.1819, 35.6797) ccw
  arc A50 (57.8176, 35.8449) -> (58.37, 37.2123) centre (41.6795, 43.1604) ccw
  arc A51 (58.8728, 37.4577) -> (58.37, 37.2123) centre (58.7468, 37.078) ccw
  line L25 (58.8728, 37.4577) -> (59.7752, 37.1583)
  spline S48 degree 3 poles (60.6415, 37.0652) (60.1488, 37.0715) (59.8677, 37.1338) (59.7752, 37.1583) knots 0 0 0 0 1 1 1 1
  spline S49 degree 3 poles (63.2169, 37.4668) (62.095, 37.1361) (61.2285, 37.0586) (60.6415, 37.0652) knots 0 0 0 0 1 1 1 1
  arc A52 (63.2169, 37.4668) -> (63.533, 38.8364) centre (41.6795, 43.1604) ccw
  spline S50 degree 3 poles (61.3934, 40.3273) (61.9249, 40.0749) (62.6698, 39.6254) (63.533, 38.8364) knots 0 0 0 0 1 1 1 1
  spline S51 degree 3 poles (60.5749, 40.6224) (60.6688, 40.6038) (60.9488, 40.5367) (61.3934, 40.3273) knots 0 0 0 0 1 1 1 1
  line L26 (60.5749, 40.6224) -> (59.6326, 40.7489)
  arc A53 (59.2883, 41.1899) -> (59.6326, 40.7489) centre (59.6859, 41.1454) ccw
  arc A54 (59.2883, 41.1899) -> (59.3912, 42.6611) centre (41.6795, 43.1604) ccw
  arc A55 (59.7935, 43.0498) -> (59.3912, 42.6611) centre (59.7911, 42.6498) ccw
  line L27 (59.7935, 43.0498) -> (60.7442, 43.044)
  spline S52 degree 3 poles (61.5969, 43.2231) (61.1264, 43.0768) (60.8398, 43.0493) (60.7442, 43.044) knots 0 0 0 0 1 1 1 1
  spline S53 degree 3 poles (63.9222, 44.4009) (62.9575, 43.7397) (62.1573, 43.3982) (61.5969, 43.2231) knots 0 0 0 0 1 1 1 1
  arc A56 (63.9222, 44.4009) -> (63.7996, 45.8011) centre (41.6795, 43.1604) ccw
  spline S54 degree 3 poles (61.304, 46.5579) (61.8875, 46.4821) (62.7348, 46.2848) (63.7996, 45.8011) knots 0 0 0 0 1 1 1 1
  spline S55 degree 3 poles (60.4344, 46.5856) (60.5294, 46.597) (60.8164, 46.6196) (61.304, 46.5579) knots 0 0 0 0 1 1 1 1
  line L28 (60.4344, 46.5856) -> (59.4991, 46.4148)
  arc A57 (59.0354, 46.7277) -> (59.4991, 46.4148) centre (59.4272, 46.8083) ccw
  arc A58 (59.0354, 46.7277) -> (58.6786, 48.1587) centre (41.6795, 43.1604) ccw
  arc A59 (58.9411, 48.6527) -> (58.6786, 48.1587) centre (59.0624, 48.2715) ccw
  line L29 (58.9411, 48.6527) -> (59.8471, 48.941)
  spline S56 degree 3 poles (60.6027, 49.3749) (60.2004, 49.0903) (59.9364, 48.9755) (59.8471, 48.941) knots 0 0 0 0 1 1 1 1
  spline S57 degree 3 poles (62.4502, 51.2135) (61.737, 50.2866) (61.0815, 49.7145) (60.6027, 49.3749) knots 0 0 0 0 1 1 1 1
  arc A60 (62.4502, 51.2135) -> (61.901, 52.5074) centre (41.6795, 43.1604) ccw
  spline S58 degree 3 poles (59.2936, 52.4559) (59.8719, 52.5641) (60.7388, 52.6383) (61.901, 52.5074) knots 0 0 0 0 1 1 1 1
  spline S59 degree 3 poles (58.458, 52.2135) (58.5449, 52.2537) (58.8108, 52.3639) (59.2936, 52.4559) knots 0 0 0 0 1 1 1 1
  line L30 (58.458, 52.2135) -> (57.6213, 51.7621)
  arc A61 (57.0836, 51.9164) -> (57.6213, 51.7621) centre (57.4313, 52.1141) ccw
  arc A62 (57.0836, 51.9164) -> (56.3021, 53.1671) centre (41.6795, 43.1604) ccw
  arc A63 (56.399, 53.718) -> (56.3021, 53.1671) centre (56.6322, 53.393) ccw
  line L31 (56.399, 53.718) -> (57.1716, 54.2722)
  spline S60 degree 3 poles (57.7562, 54.9183) (57.4615, 54.5234) (57.2458, 54.3326) (57.1716, 54.2722) knots 0 0 0 0 1 1 1 1
  spline S61 degree 3 poles (58.945, 57.2379) (58.5532, 56.1359) (58.1066, 55.3893) (57.7562, 54.9183) knots 0 0 0 0 1 1 1 1
  arc A64 (58.945, 57.2379) -> (58.0229, 58.2987) centre (41.6795, 43.1604) ccw
  spline S62 degree 3 poles (55.5591, 57.444) (56.0756, 57.7256) (56.8771, 58.0641) (58.0229, 58.2987) knots 0 0 0 0 1 1 1 1
  spline S63 degree 3 poles (54.8392, 56.9553) (54.9094, 57.0203) (55.1283, 57.2073) (55.5591, 57.444) knots 0 0 0 0 1 1 1 1
  line L32 (54.8392, 56.9553) -> (54.183, 56.2673)
  arc A65 (53.6239, 56.248) -> (54.183, 56.2673) centre (53.8935, 56.5434) ccw
  arc A66 (53.6239, 56.248) -> (52.4942, 57.196) centre (41.6795, 43.1604) ccw
  arc A67 (52.4161, 57.7499) -> (52.4942, 57.196) centre (52.7383, 57.5128) ccw
  line L33 (52.4161, 57.7499) -> (52.9797, 58.5156)
  spline S64 degree 3 poles (53.3359, 59.3108) (53.1777, 58.8441) (53.0315, 58.5961) (52.9797, 58.5156) knots 0 0 0 0 1 1 1 1
  spline S65 degree 3 poles (53.7498, 61.8842) (53.7177, 60.7151) (53.5236, 59.867) (53.3359, 59.3108) knots 0 0 0 0 1 1 1 1
  arc A68 (53.7498, 61.8842) -> (52.545, 62.6081) centre (41.6795, 43.1604) ccw
  spline S66 degree 3 poles (50.4659, 61.0339) (50.8701, 61.4614) (51.5278, 62.0309) (52.545, 62.6081) knots 0 0 0 0 1 1 1 1
  spline S67 degree 3 poles (49.9323, 60.3467) (49.9789, 60.4303) (50.1293, 60.6758) (50.4659, 61.0339) knots 0 0 0 0 1 1 1 1
  line L34 (49.9323, 60.3467) -> (49.5207, 59.4896)
  arc A69 (48.995, 59.2985) -> (49.5207, 59.4896) centre (49.1602, 59.6628) ccw
  arc A70 (48.995, 59.2985) -> (47.6276, 59.8509) centre (41.6795, 43.1604) ccw
  arc A71 (47.3822, 60.3536) -> (47.6276, 59.8509) centre (47.7619, 60.2277) ccw
  line L35 (47.3822, 60.3536) -> (47.6815, 61.256)
  spline S68 degree 3 poles (47.7747, 62.1224) (47.7684, 61.6296) (47.706, 61.3486) (47.6815, 61.256) knots 0 0 0 0 1 1 1 1
  spline S69 degree 3 poles (47.3731, 64.6977) (47.7038, 63.5759) (47.7813, 62.7094) (47.7747, 62.1224) knots 0 0 0 0 1 1 1 1
  arc A72 (47.3731, 64.6977) -> (46.0035, 65.0139) centre (41.6795, 43.1604) ccw
  spline S70 degree 3 poles (44.5126, 62.8743) (44.765, 63.4058) (45.2145, 64.1506) (46.0035, 65.0139) knots 0 0 0 0 1 1 1 1
  spline S71 degree 3 poles (44.2175, 62.0558) (44.236, 62.1497) (44.3032, 62.4296) (44.5126, 62.8743) knots 0 0 0 0 1 1 1 1
  line L36 (44.2175, 62.0558) -> (44.0909, 61.1135)
  arc A73 (43.65, 60.7692) -> (44.0909, 61.1135) centre (43.6945, 61.1667) ccw
  arc A74 (43.65, 60.7692) -> (42.1788, 60.8721) centre (41.6795, 43.1604) ccw
  arc A75 (41.7901, 61.2744) -> (42.1788, 60.8721) centre (42.1901, 61.2719) ccw
  line L37 (41.7901, 61.2744) -> (41.7959, 62.2251)
  spline S72 degree 3 poles (41.6168, 63.0778) (41.7631, 62.6073) (41.7906, 62.3207) (41.7959, 62.2251) knots 0 0 0 0 1 1 1 1
  spline S73 degree 3 poles (40.439, 65.403) (41.1002, 64.4383) (41.4417, 63.6381) (41.6168, 63.0778) knots 0 0 0 0 1 1 1 1
  arc A76 (40.439, 65.403) -> (39.0388, 65.2805) centre (41.6795, 43.1604) ccw
  spline S74 degree 3 poles (38.282, 62.7849) (38.3578, 63.3683) (38.5551, 64.2157) (39.0388, 65.2805) knots 0 0 0 0 1 1 1 1
  spline S75 degree 3 poles (38.2543, 61.9153) (38.2429, 62.0103) (38.2203, 62.2973) (38.282, 62.7849) knots 0 0 0 0 1 1 1 1
  line L38 (38.2543, 61.9153) -> (38.4251, 60.98)
  arc A77 (38.1121, 60.5163) -> (38.4251, 60.98) centre (38.0316, 60.9081) ccw
  arc A78 (38.1121, 60.5163) -> (36.6812, 60.1595) centre (41.6795, 43.1604) ccw
  arc A79 (36.1872, 60.422) -> (36.6812, 60.1595) centre (36.5683, 60.5433) ccw
  line L39 (36.1872, 60.422) -> (35.8989, 61.328)
  spline S76 degree 3 poles (35.465, 62.0836) (35.7496, 61.6813) (35.8643, 61.4172) (35.8989, 61.328) knots 0 0 0 0 1 1 1 1
  spline S77 degree 3 poles (33.6264, 63.9311) (34.5533, 63.2179) (35.1253, 62.5624) (35.465, 62.0836) knots 0 0 0 0 1 1 1 1
  arc A80 (33.6264, 63.9311) -> (32.3325, 63.3819) centre (41.6795, 43.1604) ccw
  spline S78 degree 3 poles (32.384, 60.7745) (32.2758, 61.3528) (32.2016, 62.2197) (32.3325, 63.3819) knots 0 0 0 0 1 1 1 1
  spline S79 degree 3 poles (32.6264, 59.9389) (32.5862, 60.0257) (32.476, 60.2917) (32.384, 60.7745) knots 0 0 0 0 1 1 1 1
  circle A81 centre (41.6795, 43.1604) radius 12.5
  circle A82 centre (41.6795, 43.1604) radius 5.25
  dimension "d62" = 25
  dimension "d63" = 10.5
  measures "d62" diameter of A81
  measures "d63" diameter of A82
extrude "Extrude1'''" add sketch "Sketch13" against normal blind 8 separate body contours A0 A81 makes body 4 in component "Component"
sketch "Sketch14" plane through (0, 0, 0) normal (0, 1, 0) x (1, 0, 0)
  circle A0 centre (41.6795, -43.1604) radius 5.25
extrude "Extrude1''''" add sketch "Sketch14" along normal blind -10 and the other way blind -20 separate body makes body 5 in component "Component'"